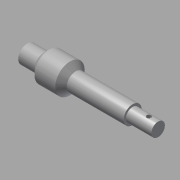
# Autodesk Inventor part: Ball Shifting Shaft
Saved by Autodesk Inventor 2013 (Build 170138000, 138)
## iProperties
Created: 2013-09-04
Part Number: Ball Shifting Shaft
Material: Steel
Document SubType Name: Modeling
Designer: grtstudent
Density: 7.85 g/cm^3
Mass: 14.2871 g
Surface Area: 11.1953 cm^2
Volume: 1.82001 cm^3
Author: grtstudent
Autodesk Inventor part; units mm, degrees
ref_plane "YZ Plane" through (0, 0, 0) normal (1, 0, 0) x (0, 1, 0)
ref_plane "XY Plane" through (0, 0, 0) normal (0, 0, 1) x (1, 0, 0)
sketch "Sketch1" plane through (0, 0, 0) normal (0, 0, 1) x (1, 0, 0)
  line L0 (51.1505, 3.175) -> (28.5454, 3.175)
  line L1 (19.2722, 5.1753) -> (17.272, 3.175)
  line L2 (26.5452, 5.1753) -> (28.5454, 3.175)
  line L3 (9.6514, 0) -> (11.5592, 3.175)
  line L4 (17.272, 3.175) -> (11.5592, 3.175)
  line L5 (26.5452, 5.1753) -> (19.2722, 5.1753)
  line L6 (9.6514, 0) -> (51.1505, 0)
  line L7 (51.1505, 3.175) -> (51.1505, 0)
  point P0 (0, 0)
  dimension "d3" = 135
  dimension "d4" = 7.2729
  dimension "d5" = 5.7128
  dimension "d8" = 59
  dimension "d9" = 135
  dimension "d10" = 41.4991
  dimension "d11" = 3.175
  dimension "d12" = 5.1753
  dimension "d13" = 3.175
  dimension "d14" = 9.6514
  constraints: 16 end point, 1 coincident, 1 horizontal, 1 horizontal alignment, 1 perpendicular, 1 point on line
  measures "d3" angle of L0 L2
  measures "d4" distance of L1.start L5.start
  measures "d5" distance of L4.start L3.end
  measures "d8" angle of L6 L3
  measures "d9" angle of L4 L1
  measures "d10" distance from line of L7 L6.start
  measures "d11" distance between parallel lines of L4 L6
  measures "d12" distance between parallel lines of L5 L6
  measures "d13" distance between parallel lines of L0 L6
  measures "d14" distance of L6.start point (0, 0)
revolve "Revolution1" add sketch "Sketch1" angle 360 about axis through (9.6514, 0, 0) along (1, 0, 0)
sketch "Sketch2" plane through (51.1505, 0, 0) normal (1, 0, 0) x (0, 0, -1)
  circle A0 centre (0, 0) radius 3.175 projected
extrude "Extrusion1" cut sketch "Sketch2" against normal blind 4.9784
sketch "Sketch5" plane through (46.1721, 0, 0) normal (1, 0, 0) x (0, 0, -1)
  circle A0 centre (0, 0) radius 3.175 projected
extrude "Extrusion4" add sketch "Sketch5" along normal blind 2.3813
sketch "Sketch6" plane through (48.5534, 0, 0) normal (1, 0, 0) x (0, 0, -1)
  circle A0 centre (0, 0) radius 3.175 projected
  circle A1 centre (0, 0) radius 2.3813
  dimension "d30" = 4.7625
  constraints: 1 centre point, 1 coincident
  measures "d30" diameter of A1
extrude "Extrusion5" add sketch "Sketch6" along normal blind 8.9472 contours A1
ref_plane "Work Plane1" through (48.5534, 2.3813, 0) normal (0, 1, 0) x (-1, 0, 0)
sketch "Sketch7" plane through (48.5534, 2.3813, 0) normal (0, 1, 0) x (-1, 0, 0)
  line L0 (-8.9471, 2.3813) -> (-8.9471, -2.3813) projected
  line L1 (0, -2.3813) -> (0, 2.3813) projected
  line L2 (-8.9471, 0) -> (0, 0) construction
  circle A0 centre (-5.7721, 0) radius 0.7937
  point P0 (48.5534, 0)
  dimension "d34" = 1.5875
  dimension "d36" = 5.7721
  constraints: 2 end point, 2 midpoint, 1 centre point, 1 point on line
  measures "d34" diameter of A0
  measures "d36" distance from line of L1 A0.centre
extrude "Extrusion6" cut sketch "Sketch7" against normal through all
body "Solid1"
